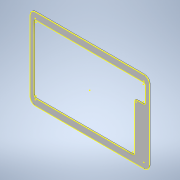
# Autodesk Inventor part: UpperAcrylicPlate
Saved by Autodesk Inventor 2022 (Build 260153000, 153)
## iProperties
Created: 2021-04-23
Part Number: UpperAcrylicPlate
Material: Generic
Document SubType Name: Modeling
Designer: Viktor
Density: 1 g/cm^3
Appearance: Default
Author: Viktor
Autodesk Inventor part; units mm, degrees
ref_plane "YZ Plane" through (0, 0, 0) normal (1, 0, 0) x (0, 1, 0)
ref_plane "XZ Plane" through (0, 0, 0) normal (0, 1, 0) x (-1, 0, 0)
ref_plane "XY Plane" through (0, 0, 0) normal (0, 0, 1) x (1, 0, 0)
sketch "Sketch1" plane through (0, 0, 0) normal (0, 0, 1) x (1, 0, 0)
  line L0 (-219.75, -149.75) -> (219.75, -149.75)
  line L1 (219.75, -149.75) -> (219.75, 149.75)
  line L2 (219.75, 149.75) -> (-219.75, 149.75)
  line L3 (-219.75, 149.75) -> (-219.75, -149.75)
  line L4 (-219.75, -149.75) -> (219.75, 149.75) construction
  line L5 (219.75, -149.75) -> (-219.75, 149.75) construction
  point P0 (0, 0)
  dimension "d0" = 439.5
  dimension "d1" = 299.5
  constraints: 12 end point, 2 midpoint, 2 parallel, 1 horizontal, 1 perpendicular
  measures "d0" distance between parallel lines of L1 L3
  measures "d1" distance between parallel lines of L0 L2
extrude "Extrusion1" add sketch "Sketch1" along normal blind 3
fillet "Fillet1" radius 20 4 edges at (219.75, 149.75, 1.5) (219.75, -149.75, 1.5) (-219.75, -149.75, 1.5) (-219.75, 149.75, 1.5)
sketch "Sketch2" plane through (0, 0, 3) normal (0, 0, 1) x (1, 0, 0)
  line L0 (-313.799, 0) -> (313.799, 0) construction
  line L1 (-199.75, -149.75) -> (199.75, -149.75) projected
  arc A0 (-219.75, -129.75) -> (-199.75, -149.75) centre (-199.75, -129.75) ccw projected
  line L2 (-219.75, 129.75) -> (-219.75, -129.75) projected
  arc A1 (-199.75, 149.75) -> (-219.75, 129.75) centre (-199.75, 129.75) ccw projected
  line L3 (199.75, 149.75) -> (-199.75, 149.75) projected
  arc A2 (219.75, 129.75) -> (199.75, 149.75) centre (199.75, 129.75) ccw projected
  line L4 (219.75, -129.75) -> (219.75, 129.75) projected
  arc A3 (199.75, -149.75) -> (219.75, -129.75) centre (199.75, -129.75) ccw projected
  line L5 (199.75, -134.75) -> (-199.75, -134.75)
  arc A4 (-204.75, -129.75) -> (-199.75, -134.75) centre (-199.75, -129.75) ccw
  line L6 (-204.75, -129.75) -> (-204.75, 129.75)
  arc A5 (-199.75, 134.75) -> (-204.75, 129.75) centre (-199.75, 129.75) ccw
  line L7 (-199.75, 134.75) -> (199.75, 134.75)
  arc A6 (204.75, 129.75) -> (199.75, 134.75) centre (199.75, 129.75) ccw
  line L8 (204.75, 129.75) -> (204.75, -129.75)
  arc A7 (199.75, -134.75) -> (204.75, -129.75) centre (199.75, -129.75) ccw
  line L9 (204.75, 55.25) -> (165.25, 55.25)
  line L10 (165.25, 55.25) -> (165.25, -134.75)
  line L11 (165.25, -134.75) -> (204.75, -134.75)
  line L12 (204.75, -134.75) -> (204.75, 55.25)
  dimension "d7" = 15
  dimension "d8" = 370
  dimension "d9" = 190
  constraints: 16 end point, 8 point on circle, 4 centre point, 2 parallel, 2 point on line, 1 horizontal, 1 perpendicular, 7 other
  measures "d7" distance between parallel lines of L1 L5
  measures "d8" distance between parallel lines of L6 L10
  measures "d9" distance between parallel lines of L5 L9
extrude "Extrusion2" cut sketch "Sketch2" against normal through all contours L5 A4 L6 A5 L7 A6 L8 L9 L10
fillet "Fillet2" radius 7 3 edges at (204.75, 55.25, 1.5) (165.25, 55.25, 1.5) (165.25, -134.75, 1.5)
sketch "Sketch4" plane through (0, 0, 3) normal (0, 0, 1) x (1, 0, 0)
  line L0 (165.25, 48.25) -> (165.25, -127.75) projected
  line L1 (165.25, -124.75) -> (-206.75, -124.75)
  line L2 (-206.75, -124.75) -> (-206.75, -134.75)
  line L3 (-206.75, -134.75) -> (165.25, -134.75)
  line L4 (165.25, -134.75) -> (165.25, -124.75)
  line L5 (-206.75, 134.75) -> (204.75, 134.75)
  line L6 (204.75, 134.75) -> (204.75, 124.75)
  line L7 (204.75, 124.75) -> (-206.75, 124.75)
  line L8 (-206.75, 124.75) -> (-206.75, 134.75)
  line L9 (-199.75, 134.75) -> (199.75, 134.75) projected
  line L10 (158.25, -134.75) -> (-199.75, -134.75) projected
  point P0 (0, 0)
  point P1 (-1, 134.75)
  point P2 (204.75, 129.75)
  point P3 (-20.75, -134.75)
  point P4 (165.25, -127.75)
  dimension "d13" = 10
  dimension "d14" = 10
  constraints: 16 end point, 4 midpoint, 4 parallel, 3 point on line, 2 horizontal, 2 perpendicular
  measures "d13" distance between parallel lines of L5 L7
  measures "d14" distance between parallel lines of L3 L1
extrude "Extrusion3" add sketch "Sketch4" against normal up to surface (3 mm away)
fillet "Fillet3" radius 7 4 edges at (204.75, 124.75, 1.5) (-204.75, 124.75, 1.5) (-204.75, -124.75, 1.5) (165.25, -124.75, 1.5)
sketch "Sketch5" plane through (0, 0, 3) normal (0, 0, 1) x (1, 0, 0)
  line L0 (204.75, 117.75) -> (204.75, 62.25) projected
  arc A0 (197.75, 55.25) -> (204.75, 62.25) centre (197.75, 62.25) ccw projected
  line L1 (197.75, 55.25) -> (172.25, 55.25) projected
  arc A1 (172.25, 55.25) -> (165.25, 48.25) centre (172.25, 48.25) ccw projected
  line L2 (165.25, 48.25) -> (165.25, -117.75) projected
  arc A2 (158.25, -124.75) -> (165.25, -117.75) centre (158.25, -117.75) ccw projected
  line L3 (158.25, -124.75) -> (-197.75, -124.75) projected
  arc A3 (-204.75, -117.75) -> (-197.75, -124.75) centre (-197.75, -117.75) ccw projected
  line L4 (-204.75, -117.75) -> (-204.75, 117.75) projected
  arc A4 (-197.75, 124.75) -> (-204.75, 117.75) centre (-197.75, 117.75) ccw projected
  line L5 (-197.75, 124.75) -> (197.75, 124.75) projected
  arc A5 (204.75, 117.75) -> (197.75, 124.75) centre (197.75, 117.75) ccw projected
  arc A6 (-199.75, 149.75) -> (-219.75, 129.75) centre (-199.75, 129.75) ccw projected
  line L6 (-219.75, 129.75) -> (-219.75, -129.75) projected
  arc A7 (-219.75, -129.75) -> (-199.75, -149.75) centre (-199.75, -129.75) ccw projected
  line L7 (-199.75, -149.75) -> (199.75, -149.75) projected
  arc A8 (199.75, -149.75) -> (219.75, -129.75) centre (199.75, -129.75) ccw projected
  line L8 (219.75, -129.75) -> (219.75, 129.75) projected
  arc A9 (219.75, 129.75) -> (199.75, 149.75) centre (199.75, 129.75) ccw projected
  line L9 (199.75, 149.75) -> (-199.75, 149.75) projected
  point P0 (0, 0)
equation "\"d14\" = d13"
body "Solid1"
